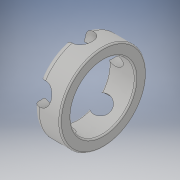
# Autodesk Inventor part: 040400DR-22-H4W(0.5)3_cage
Saved by Autodesk Inventor 2024 (Build 280153000, 153)
## iProperties
Created: 2023-06-17
Part Number: 040400DR-22-H4W(0.5)3_cage
Material: Generic
Catalog Web Link: www.cadenas.de
Description: DR-H cage-D-Series bearings
Vendor: TOKBEARING
Document SubType Name: Modeling
Designer: psAdmin
Manufacturer: TOKBEARING
Mass: 8300 g
Surface Area: 4.67681 cm^2
Volume: 0.256784 cm^3
Density: 1 g/cm^3
Appearance: PSOLRGB-175-175-175
Category: PARTsolutions
Company: TOKBEARING
PSOL_IDENT_0: {$CADENAS_DATA/23d-libs/tok_bearing/d_series_bearings/dr_h/dr_h_cage.prj},197 {VTYP=3D},{NB=040400DR
PSOL_IDENT_1: -22-H4W(0.5)3_cage},{LINA=040400DR-22-H4W(0.5)3_cage},{NN=DR-H cage},{DATE=16.12.2020 00:38:04},{GEO
PSOL_IDENT_2: MDATE=03.12.2012 14:40:00},{VERSION=},{LINEID=1750},{WBVAR=},{WBNUMERIC=}  {NB=040400DR-22-H4W(0.5)3
PSOL_IDENT_3: _cage},{LINA=040400DR-22-H4W(0.5)3_cage},{KT=DUMMY},{IDNR=},{CODE=040400},{PN=DR-22-H4W(0.5)3},{D=22
PSOL_IDENT_4: },{SD=4.0},{W=7},{W1=0.5},{W1X=0.500},{W2=3},{W2X=3.000},{LOAD=196 (20)},{TYPE=12},{QTY=1.000},{GW=8
PSOL_IDENT_5: .3},{BD=3.78},{OP=40.2862},{N=5},{R=6.415},{GP=3.64}
NB: 040400DR-22-H4W(0.5)3_cage
NN: DR-H cage
NT: D-Series bearings
NBSYN: $CODE.$PN._cage
LINA: 040400DR-22-H4W(0.5)3_cage
CATALOG: TOK, Inc
CODE: 040400
PN: DR-22-H4W(0.5)3
D: 22
SD: 4
W: 7
W1: 0.5
W2: 3
LOAD: 196 (20)
TYPE: 12
QTY: 1.000
GW: 8.3
SUPPLIER: TOKBEARING
ARTICLENO: 040400DR-22-H4W(0.5)3_cage
BOMINFO: 040400DR-22-H4W(0.5)3_cage
CREATOR: CADENAS GmbH
Title: 040400DR-22-H4W(0.5)3_cage
Author: Cadenas PARTsolutions
Comments: D-Series bearings
Autodesk Inventor part; units mm, degrees
note: some values were not read from the file. Chosen so that the rebuilt part matches the saved one: pattern direction of "Circular Pattern1".
sketch "Sketch_1" plane through (0, 0, 0) normal (0, 0, 1) x (1, 0, 0)
  line L0 (7.5, 0) -> (2.95, 0)
  arc A0 (2.95, 5.7033) -> (3.1833, 5.47) centre (3.1833, 5.7033) ccw
  line L1 (3.1833, 5.47) -> (7.2667, 5.47)
  arc A1 (7.2667, 5.47) -> (7.5, 5.7033) centre (7.2667, 5.7033) ccw
  line L2 (7.5, 5.7033) -> (7.5, 7.1267)
  arc A2 (7.5, 7.1267) -> (7.2667, 7.36) centre (7.2667, 7.1267) ccw
  line L3 (7.2667, 7.36) -> (3.95, 7.36)
  arc A3 (3.95, 7.36) -> (2.95, 6.36) centre (3.95, 6.36) ccw
  line L4 (2.95, 6.36) -> (2.95, 5.7033)
  constraints: 10 end point, 8 point on circle, 4 centre point
revolve "Revolution1" add sketch "Sketch_1" angle 360 about axis through (7.5, 0, 0) along (1, 0, 0)
sketch "Sketch_2" plane through (4, 0, 0) normal (1, 0, 0) x (0, 0, -1)
  line L0 (0, 8.305) -> (0, 4.525)
  arc A0 (0, 8.305) -> (0, 4.525) centre (0, 6.415) ccw
  line L1 (0, 8.305) -> (0, 4.525)
  constraints: 4 end point, 2 point on circle, 1 centre point
revolve "Revolution2" cut sketch "Sketch_2" angle 360 about axis through (4, 8.305, 0) along (0, 1, 0)
pattern_circular "Circular Pattern1" count 5 over 360 about axis through (4, 0, 0) along (1, 0, 0) of "Revolution2"
ref_plane "Cage_OR_XY" through (0, 0, 0) normal (1, 0, 0) x (0, 0, -1)
ref_plane "Cage_OR_YZ" through (0, 0, 0) normal (0, 0, -1) x (0, 1, 0)
ref_plane "Cage_OR_ZX" through (0, 0, 0) normal (0, 1, 0) x (1, 0, 0)
body "Solid1"
